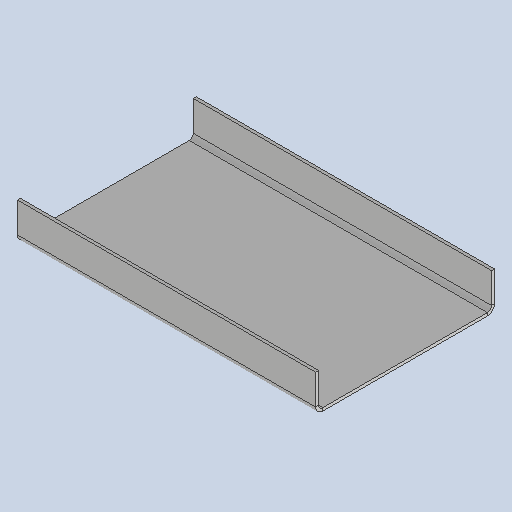
# Autodesk Inventor part: TRM 037 box 2
Saved by Autodesk Inventor 2025 (Build 290162010, 162A)
## iProperties
Created: 2024-08-07
Part Number: TRM 037 box 2
Material: AISI 304
Document SubType Name: Sheet Metal
Designer: user
Stock Number: ТРМ 026 правый борт успокоитель
Mass: 522.701 g
Surface Area: 665.635 cm^2
Volume: 65.1124 cm^3
Density: 8.02768 g/cm^3
Flat Pattern Width: 20 cm
Flat Pattern Length: 16.2404 cm
Flat Pattern Area: 324.808 cm^2
Sheet Metal Rule: AISI304 2mm Die16
Sheet Metal Width: 200.000 mm
Sheet Metal Length: 162.404 mm
Sheet Metal Area: 32480.796 mm^2
Appearance: Default
Author: pokla
Autodesk Inventor part; units mm, degrees
ref_plane "YZ Plane" through (0, 0, 0) normal (1, 0, 0) x (0, 1, 0)
ref_plane "XZ Plane" through (0, 0, 0) normal (0, 1, 0) x (-1, 0, 0)
ref_plane "XY Plane" through (0, 0, 0) normal (0, 0, 1) x (1, 0, 0)
sketch "Sketch1" plane through (0, 0, 0) normal (0, 0, 1) x (1, 0, 0)
  line L0 (-100, -60) -> (100, -60)
  line L1 (100, -60) -> (100, 60)
  line L2 (100, 60) -> (-100, 60)
  line L3 (-100, 60) -> (-100, -60)
  line L4 (-100, -60) -> (100, 60) construction
  line L5 (100, -60) -> (-100, 60) construction
  point P0 (0, 0)
  dimension "d0" = 200
  dimension "d1" = 120
  measures "d0" distance of L2.end L1.end
  measures "d1" distance of L1.end L0.end
extrude "Plate1" add sketch "Sketch1" along normal blind 2
sketch "Sketch2" plane through (0, 0, 0) normal (0, 0, -1) x (-1, 0, 0)
  line L0 (-80, 40) -> (120, 40) construction
  line L1 (120, 40) -> (120, 20) construction
  line L2 (120, 20) -> (-80, 20) construction
  line L3 (-80, 20) -> (-80, 40) construction
  line L4 (-100, 60) -> (100, 60) projected
  line L5 (-100, -60) -> (-100, 60) projected
  point P0 (0, 0)
  point P1 (-48, 100)
  point P2 (-50, 98)
  dimension "d6" = 200
  dimension "d9" = 20
  dimension "d10" = 20
  dimension "d11" = 20
  constraints: 4 other
  measures "d6" distance of L0.start L0.end
  measures "d9" distance of L0.end L1.end
  measures "d11" length of L3
mark "Mark1"
sketch "Sketch3" plane through (100, 58, 0) normal (0, 1, 0) x (-1, 0, 0)
  line L0 (200, 0) -> (0, 0)
  line L1 (0, 0) -> (0, -25)
  line L2 (0, -25) -> (200, -25)
  line L3 (200, -25) -> (200, 0)
  constraints: 6 end point, 1 horizontal, 1 perpendicular, 1 vertical
edge flange "Flange1" height 25 angle 90 thickness 2 bend radius 2.75 thickness toward (0, 1, 0) relief round relief width 2 relief depth 1 corner gap 2.75 corner form 0 edges at (0, 60, 0) (0, -60, 0) wall of the first edge with corners at (-100, 58, 0) (100, 58, 0) (100, 58, 25) (-100, 58, 25)
bend "Bend1"
corner "Corner1"
equation "\"d2\" = Thickness"
equation "\"d12\" = BendReliefWidth"
equation "\"d13\" = BendReliefDepth"
equation "\"d14\" = MinimumRemnant"
equation "\"d15\" = TransitionRadius"
equation "\"d18\" = BendRadius"
equation "\"d19\" = CornerReliefSize"
equation "\"d20\" = GapSize"
equation "\"d21\" = JacobiRadiusSize"
equation "\"BendReliefWidth\" = Thickness"
equation "\"BendReliefDepth\" = 0.5 * Thickness"
equation "\"CornerReliefSize\" = 4 * Thickness"
equation "\"MinimumRemnant\" = 2 * Thickness"
equation "\"TransitionRadius\" = BendRadius"
equation "\"JacobiRadiusSize\" = BendRadius"
equation "\"GapSize\" = Thickness"
equation "\"Thickness\" = 2"
equation "\"BendRadius\" = 2.75"
body "Solid1"
